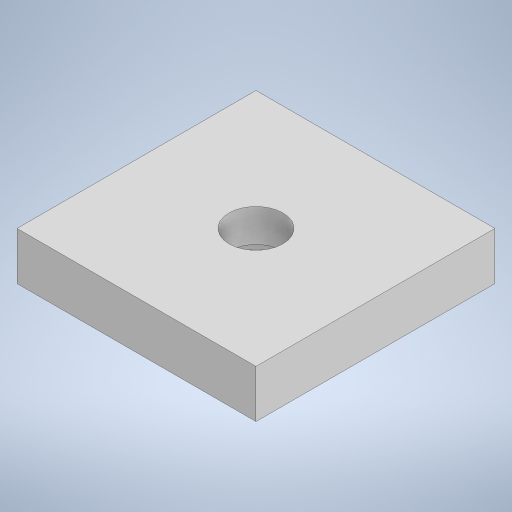
# Autodesk Inventor part: Fissante
Saved by Autodesk Inventor 2024 (Build 280153000, 153)
## iProperties
Created: 2024-01-15
Part Number: Fissante
Material: Generico
Document SubType Name: Modeling
Designer: Leonardo
Density: 1 g/cm^3
Appearance: Default
Author: Leonardo
Autodesk Inventor part; units mm, degrees
ref_plane "YZ Plane" through (0, 0, 0) normal (1, 0, 0) x (0, 1, 0)
ref_plane "XZ Plane" through (0, 0, 0) normal (0, 1, 0) x (-1, 0, 0)
ref_plane "XY Plane" through (0, 0, 0) normal (0, 0, 1) x (1, 0, 0)
sketch "Schizzo1" plane through (0, 0, 0) normal (0, 1, 0) x (-1, 0, 0)
  circle A0 centre (0, 0) radius 1
  line L0 (10, 0) -> (10, -10)
  line L1 (10, -10) -> (0, -10)
  line L2 (-10, 0) -> (-10, -10)
  line L3 (-10, -10) -> (0, -10)
  line L4 (10, 0) -> (10, 10)
  line L5 (10, 10) -> (-10, 10)
  line L6 (-10, 10) -> (-10, 0)
  dimension "d2" = 2
  dimension "d12" = 10
  dimension "d13" = 10
  dimension "d14" = 10
  dimension "d15" = 10
  constraints: 14 end point, 2 perpendicular, 1 centre point, 1 point on line, 1 vertical
  measures "d2" diameter of A0
  measures "d12" distance of L0.end L1.end
  measures "d13" distance of L0.start L0.end
  measures "d14" distance of L3.end L2.end
  measures "d15" distance of L0.start L4.end
extrude "Estrusione2" add sketch "Schizzo1" along normal blind 4
sketch "Schizzo3" plane through (0, 0, 0) normal (0, -1, 0) x (1, 0, 0)
  point P0 (0, 0)
  point P1 (0, 0)
  constraints: 1 coincident
hole "Foro2" at (0, 0, 0) direction (0, 1, 0) diameter 4.5 depth 8 countersink diameter 7 countersink angle 90
